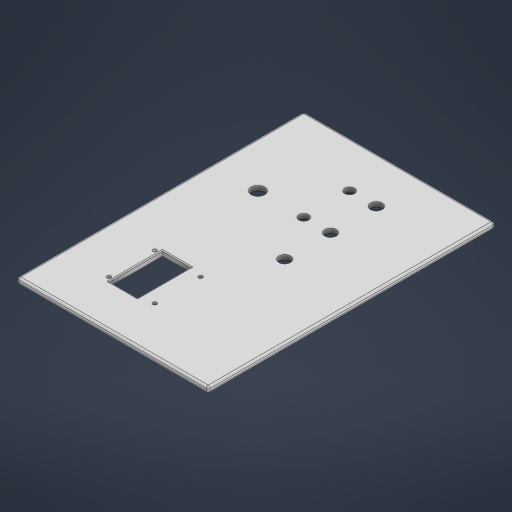
# Autodesk Inventor part: ecu-box-lid
Saved by Autodesk Inventor 2024.2 (Build 282272000, 272)
## iProperties
Created: 2025-06-20
Part Number: ecu-box-lid
Material: Generic
Document SubType Name: Modeling
Designer: Moe
Density: 1 g/cm^3
Appearance: Default
Author: Moe
Autodesk Inventor part; units mm, degrees
ref_plane "YZ Plane" through (0, 0, 0) normal (1, 0, 0) x (0, 1, 0)
ref_plane "XZ Plane" through (0, 0, 0) normal (0, 1, 0) x (-1, 0, 0)
ref_plane "XY Plane" through (0, 0, 0) normal (0, 0, 1) x (1, 0, 0)
sketch "Sketch1" plane through (0, 0, 0) normal (0, 1, 0) x (-1, 0, 0)
  line L0 (0, 0) -> (100, 0)
  line L1 (100, 0) -> (100, -150)
  line L2 (100, -150) -> (0, -150)
  line L3 (0, -150) -> (0, 0)
  dimension "d0" = 100
  dimension "d1" = 150
  constraints: 8 end point, 2 parallel, 1 horizontal, 1 perpendicular
  measures "d0" distance of L1.end L2.end
  measures "d1" distance of L0.end L1.end
extrude "Extrusion1" add sketch "Sketch1" along normal blind 3
sketch "Sketch2" plane through (0, 0, 0) normal (0, -1, 0) x (1, 0, 0)
  line L0 (0, -150) -> (-100, -150) projected
  line L1 (0, 0) -> (0, -150) projected
  line L2 (-100, 0) -> (0, 0) projected
  line L3 (-100, -150) -> (-100, 0) projected
  line L4 (-5.25, -3.25) -> (-94.75, -3.25)
  line L5 (-96.75, -5.25) -> (-96.75, -144.75)
  line L6 (-94.75, -146.75) -> (-5.25, -146.75)
  line L7 (-3.25, -144.75) -> (-3.25, -5.25)
  arc A0 (-3.25, -5.25) -> (-5.25, -3.25) centre (-5.25, -5.25) ccw
  arc A1 (-94.75, -3.25) -> (-96.75, -5.25) centre (-94.75, -5.25) ccw
  arc A2 (-96.75, -144.75) -> (-94.75, -146.75) centre (-94.75, -144.75) ccw
  arc A3 (-5.25, -146.75) -> (-3.25, -144.75) centre (-5.25, -144.75) ccw
  line L8 (-8.25, -6.25) -> (-91.75, -6.25)
  line L9 (-93.75, -8.25) -> (-93.75, -141.75)
  line L10 (-91.75, -143.75) -> (-8.25, -143.75)
  line L11 (-6.25, -141.75) -> (-6.25, -8.25)
  arc A4 (-6.25, -8.25) -> (-8.25, -6.25) centre (-8.25, -8.25) ccw
  arc A5 (-8.25, -143.75) -> (-6.25, -141.75) centre (-8.25, -141.75) ccw
  arc A6 (-93.75, -141.75) -> (-91.75, -143.75) centre (-91.75, -141.75) ccw
  arc A7 (-91.75, -6.25) -> (-93.75, -8.25) centre (-91.75, -8.25) ccw
  point P0 (-3.25, -3.25)
  point P1 (-96.75, -146.75)
  point P2 (-96.75, -3.25)
  point P3 (-3.25, -146.75)
  point P4 (-50, -143.75)
  dimension "d4" = 3.25
  dimension "d5" = 3.25
  dimension "d6" = 3.25
  dimension "d7" = 3.25
  dimension "d10" = 2
  dimension "d12" = 3
  dimension "d13" = 3
  dimension "d14" = 3
  dimension "d15" = 3
  dimension "d16" = 2
  constraints: 16 end point, 16 point on circle, 16 tangent, 8 centre point, 8 point on line, 6 equal radius, 4 parallel, 2 horizontal, 2 perpendicular, 1 midpoint
  measures "d4" distance between parallel lines of L1 L7
  measures "d5" distance between parallel lines of L3 L5
  measures "d6" distance between parallel lines of L2 L4
  measures "d7" distance between parallel lines of L0 L6
  measures "d10" radius of A0
  measures "d12" distance between parallel lines of L7 L11
  measures "d13" distance between parallel lines of L4 L8
  measures "d14" distance between parallel lines of L5 L9
  measures "d15" distance from line of L6 point (-50, -143.75)
  measures "d16" radius of A4
extrude "Extrusion2" add sketch "Sketch2" along normal blind 3 contours A0 L7 A3 L6 A2 L5 A1 L4
fillet "Fillet1" radius 1 20 edges at (-50, 0, 0) (0, 1.5, 0) (0, 0, -75) (0, 3, -75) (-50, 3, 0) (-3.8358, -3, -3.8358) (-50, -3, -3.25) (-96.1642, -3, -3.8358) (-96.75, -3, -75) (-96.1642, -3, -146.1642) (-50, -3, -146.75) (-3.8358, -3, -146.1642) (-3.25, -3, -75) (0, 1.5, -150) (-50, 3, -150) (-50, 0, -150) (-100, 3, -75) (-100, 1.5, -150) (-100, 0, -75) (-100, 1.5, 0)
sketch "Sketch4" plane through (0, 3, 0) normal (0, 1, 0) x (1, 0, 0)
  circle A0 centre (-52, 102) radius 2.5
  circle A1 centre (-51.9995, 126) radius 2.5
  circle A2 centre (-38, 78) radius 3
  circle A3 centre (-38, 102) radius 3
  circle A4 centre (-37.9995, 126) radius 3
  circle A5 centre (-76, 102) radius 3.5
  circle A6 centre (-76, 24) radius 1
  circle A7 centre (-76, 48) radius 1
  circle A8 centre (-52, 23.9998) radius 1
  circle A9 centre (-52, 47.9998) radius 1
  line L0 (-100, 149) -> (-100, 1) projected
  line L1 (0, 1) -> (0, 149) projected
  line L2 (-1, 150) -> (-99, 150) projected
  line L3 (-99, 0) -> (-1, 0) projected
  line L4 (-74, 22) -> (-59, 22)
  line L5 (-59, 22) -> (-59, 50)
  line L6 (-59, 50) -> (-74, 50)
  line L7 (-74, 50) -> (-74, 22)
  point P0 (0, 0)
  dimension "d19" = 5
  dimension "d20" = 5
  dimension "d21" = 6
  dimension "d22" = 6
  dimension "d23" = 6
  dimension "d24" = 7
  dimension "d25" = 2
  dimension "d26" = 2
  dimension "d27" = 2
  dimension "d28" = 2
  dimension "d29" = 24
  dimension "d30" = 24
  dimension "d31" = 24
  dimension "d32" = 24
  dimension "d33" = 33.941
  dimension "d34" = 0
  dimension "d35" = 24
  dimension "d36" = 24
  dimension "d37" = 14
  dimension "d38" = 14
  dimension "d39" = 24
  dimension "d40" = 14
  dimension "d41" = 24
  dimension "d42" = 24
  dimension "d43" = 38
  dimension "d46" = 48
  dimension "d47" = 24
  dimension "d48" = 24
  dimension "d49" = 15
  dimension "d50" = 28
  dimension "d51" = 2
  dimension "d52" = 2
  dimension "d53" = 2
  constraints: 10 centre point, 8 end point, 2 parallel, 1 horizontal, 1 perpendicular
  measures "d19" diameter of A0
  measures "d20" diameter of A1
  measures "d21" diameter of A2
  measures "d22" diameter of A3
  measures "d23" diameter of A4
  measures "d24" diameter of A5
  measures "d25" diameter of A6
  measures "d26" diameter of A7
  measures "d27" diameter of A8
  measures "d28" diameter of A9
  measures "d29" distance of A7.centre A9.centre
  measures "d30" distance of A8.centre A9.centre
  measures "d31" distance of A8.centre A6.centre
  measures "d32" distance of A7.centre A6.centre
  measures "d33" distance of A9.centre A6.centre
  measures "d34" horizontal distance of A7.centre A6.centre
  measures "d35" distance of A3.centre A2.centre
  measures "d36" distance of A4.centre A3.centre
  measures "d37" distance of A0.centre A3.centre
  measures "d38" distance of A1.centre A4.centre
  measures "d39" distance of A1.centre A0.centre
  measures "d40" horizontal distance of A0.centre A2.centre
  measures "d41" distance of A5.centre A0.centre
  measures "d42" distance from line of L0 A5.centre
  measures "d43" distance from line of L1 A3.centre
  measures "d46" distance from line of L2 A0.centre
  measures "d47" distance from line of L3 A6.centre
  measures "d48" distance from line of L0 A6.centre
  measures "d49" distance of L6.end L5.end
  measures "d50" distance of L5.end L4.end
  measures "d51" distance from line of A6.centre L4
  measures "d52" distance from line of A7.centre L6
  measures "d53" distance from line of A6.centre L7
extrude "Extrusion4" cut sketch "Sketch4" against normal blind 10
fillet "Fillet2" radius 0.5 14 edges at (-74, 3, -36) (-74, 0, -36) (-66.5, 0, -50) (-66.5, 3, -50) (-59, 0, -36) (-59, 3, -36) (-66.5, 0, -22) (-66.5, 3, -22) (-41, 0, -78) (-79.5, 0, -102) (-54.5, 0, -102) (-41, 0, -102) (-54.4995, 0, -126) (-40.9995, 0, -126)
body "Solid1"
